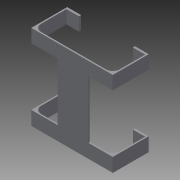
# Autodesk Inventor part: tapa
Saved by Autodesk Inventor 2013 (Build 170138000, 138)
## iProperties
Created: 2013-05-01
Part Number: tapa
Material: Generic
Document SubType Name: Modeling
Designer: otrab
Density: 1 g/cm^3
Author: otrab
Autodesk Inventor part; units mm, degrees
ref_plane "YZ Plane" through (0, 0, 0) normal (1, 0, 0) x (0, 1, 0)
ref_plane "XZ Plane" through (0, 0, 0) normal (0, 1, 0) x (-1, 0, 0)
ref_plane "XY Plane" through (0, 0, 0) normal (0, 0, 1) x (1, 0, 0)
sketch "Sketch1" plane through (0, 0, 0) normal (0, 1, 0) x (-1, 0, 0)
  line L0 (-29.5, -39) -> (29.5, -39)
  line L1 (29.5, -39) -> (29.5, 39)
  line L2 (29.5, 39) -> (-29.5, 39)
  line L3 (-29.5, 39) -> (-29.5, -39)
  line L4 (-29.5, -39) -> (29.5, 39) construction
  line L5 (29.5, -39) -> (-29.5, 39) construction
  point P0 (0, 0)
  dimension "d0" = 59
  dimension "d2" = 78
  constraints: 12 end point, 2 midpoint, 2 parallel, 1 horizontal, 1 perpendicular
  measures "d0" distance of L1.end L2.end
  measures "d2" distance of L2.end L0.start
extrude "Extrusion1" add sketch "Sketch1" along normal blind 1
sketch "Sketch2" plane through (0, 1, 0) normal (0, 1, 0) x (1, 0, 0)
  line L0 (29.5, 39) -> (-29.5, 39) projected
  line L1 (-29.5, 39) -> (-29.5, -39) projected
  line L2 (-29.5, -39) -> (29.5, -39) projected
  line L3 (-29.5, 39) -> (-28.5, 39)
  line L4 (-28.5, 39) -> (-28.5, -39)
  line L5 (-29.5, -39) -> (-28.5, -39)
  line L6 (-29.5, -39) -> (-29.5, 39)
  line L7 (0, 46.5401) -> (0, -49.8176) construction
  line L8 (29.5, 39) -> (29.5, -39)
  line L9 (29.5, 39) -> (28.5, 39)
  line L10 (28.5, 39) -> (28.5, -39)
  line L11 (29.5, -39) -> (28.5, -39)
  line L12 (29.5, -39) -> (29.5, 39)
  point P0 (0, 0)
  dimension "d5" = 1
  constraints: 20 end point, 3 perpendicular, 2 point on line, 2 symmetric about line, 1 parallel
  measures "d5" distance of L0.end L3.end
extrude "Extrusion2" add sketch "Sketch2" along normal blind 25 contours L8 L2 L10 L0 | L4 L2 L1 L0
fillet "Fillet1" radius 5 1 edges at (-28.5, 1, 0)
mirror "Mirror1" about plane through (0, 0, 0) normal (1, 0, 0) of "Fillet1"
sketch "Sketch3" plane through (-29.5, 0, -39) normal (-1, 0, 0) x (0, 0, 1)
  line L0 (0, 0) -> (78, 0) projected
  line L1 (78, 26) -> (69.75, 26) construction
  line L2 (69.75, 26) -> (69.75, 24.5)
  line L3 (69.75, 24.5) -> (59.75, 24.5)
  line L4 (59.75, 24.5) -> (59.75, 26)
  line L5 (69.75, 26) -> (59.75, 26)
  line L6 (59.75, 26) -> (69.75, 26)
  point P0 (39, 0)
  dimension "d9" = 8.25
  dimension "d10" = 1.5
  dimension "d11" = 10
  constraints: 12 end point, 1 parallel, 1 perpendicular
  measures "d9" distance of L1.start L1.end
  measures "d10" distance of L1.end L2.end
  measures "d11" distance of L2.end L3.end
extrude "Extrusion3" add sketch "Sketch3" against normal blind 10
mirror "Mirror3" about plane through (0, 0, 0) normal (0, 0, 1) of "Extrusion3"
mirror "Mirror4" about plane through (0, 0, 0) normal (1, 0, 0) of "Extrusion3", "Mirror3"
sketch "Sketch4" plane through (-29.5, 0, -39) normal (-1, 0, 0) x (0, 0, 1)
  line L0 (0, 26) -> (78, 26) projected
  line L1 (39, 26) -> (47, 26)
  line L2 (39, 26) -> (31, 26)
  line L3 (31, 26) -> (31, 12)
  line L4 (31, 12) -> (47, 12)
  line L5 (47, 12) -> (47, 26)
  point P0 (39, 0)
  dimension "d14" = 8
  dimension "d15" = 8
  dimension "d16" = 14
  constraints: 10 end point, 2 perpendicular, 2 point on line, 1 midpoint, 1 parallel
  measures "d14" distance of L1.start L1.end
  measures "d15" distance of L1.start L2.end
  measures "d16" distance of L2.end L3.end
extrude "Extrusion4" cut sketch "Sketch4" against normal up to surface (1 mm away)
mirror "Mirror5" about plane through (0, 0, 0) normal (1, 0, 0) of "Extrusion4"
sketch "Sketch6" plane through (0, 26, 0) normal (0, 1, 0) x (1, 0, 0)
  line L0 (-30.2809, -30.75) -> (31.8564, -30.75)
  line L1 (31.8564, -30.75) -> (31.8564, -41.1164)
  line L2 (31.8564, -41.1164) -> (-30.2809, -41.1164)
  line L3 (-30.2809, -41.1164) -> (-30.2809, -30.75)
  line L4 (-30.2809, 39.7218) -> (31.1002, 39.7218)
  line L5 (31.1002, 39.7218) -> (31.1002, 30.6512)
  line L6 (31.1002, 30.6512) -> (-30.2809, 30.6512)
  line L7 (-30.2809, 30.6512) -> (-30.2809, 39.7218)
  line L8 (-30.2809, 20.6535) -> (-10.2809, 20.6535)
  line L9 (-10.2809, 20.6535) -> (-10.2809, -21.1154)
  line L10 (-10.2809, -21.1154) -> (-30.2809, -21.1154)
  line L11 (-30.2809, -21.1154) -> (-30.2809, 20.6535)
  line L12 (31.8564, -21.1154) -> (11.8564, -21.1154)
  line L13 (11.8564, -21.1154) -> (11.8564, 20.6535)
  line L14 (11.8564, 20.6535) -> (31.8564, 20.6535)
  line L15 (31.8564, 20.6535) -> (31.8564, -21.1154)
  point P0 (0, 0)
  dimension "d26" = 20
  dimension "d27" = 20
  constraints: 32 end point, 8 parallel, 4 horizontal, 4 perpendicular
  measures "d26" distance of L9.end L10.end
  measures "d27" distance of L13.end L14.end
extrude "Extrusion6" cut sketch "Sketch6" against normal through all
body "Solid1"
